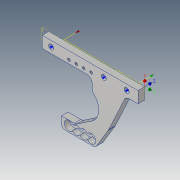
# Autodesk Inventor part: Extruder bracket
Saved by Autodesk Inventor 2019 (Build 230136000, 136)
## iProperties
Created: 2018-10-20
Part Number: Extruder bracket
Material: Aluminum 6061
Document SubType Name: Modeling
Designer: LillaHunden
Density: 2.7 g/cm^3
Appearance: Aluminum - Flat
Mass: 27.8066 g
Surface Area: 65.7368 cm^2
Volume: 10.2987 cm^3
Author: LillaHunden
Autodesk Inventor part; units mm, degrees
ref_plane "YZ Plane" through (0, 0, 0) normal (1, 0, 0) x (0, 1, 0)
ref_plane "XZ Plane" through (0, 0, 0) normal (0, 1, 0) x (-1, 0, 0)
ref_plane "XY Plane" through (0, 0, 0) normal (0, 0, 1) x (1, 0, 0)
sketch "Sketch3" plane through (0, 0, 0) normal (0, 0, 1) x (1, 0, 0)
  line L0 (-29.6423, -32.0618) -> (11.629, -32.0618)
  line L1 (11.629, -32.0618) -> (11.629, 19.8316)
  line L2 (11.629, 19.8316) -> (37.4023, 19.8316)
  line L3 (37.4023, 19.8316) -> (37.4023, 29.8316)
  line L4 (37.4023, 29.8316) -> (-52.693, 29.8316)
  line L5 (-52.693, 29.8316) -> (-52.693, 19.8316)
  line L6 (-52.693, 19.8316) -> (-2.6589, 19.8316)
  line L7 (-2.6589, 19.8316) -> (-2.6589, -22.8391)
  line L8 (-2.6589, -22.8391) -> (-29.6423, -22.8391)
  line L9 (-29.6423, -22.8391) -> (-29.6423, -32.0618)
  line L10 (37.4023, 19.8316) -> (-46.3977, 19.8316) projected
  point P0 (0, 0)
  constraints: 20 end point, 9 perpendicular, 1 horizontal, 1 horizontal alignment, 1 point on line
extrude "Extrusion3" add sketch "Sketch3" along normal blind 6
sketch "Sketch4" plane through (0, 0, 6) normal (0, 0, 1) x (1, 0, 0)
  circle A0 centre (-10.7483, -2.0987) radius 3.15 construction
  circle A1 centre (-10.7483, -2.0987) radius 13.7506
  point P0 (0, 0)
  constraints: 1 centre point, 1 coincident
extrude "Extrusion4" cut sketch "Sketch4" against normal through all
sketch "Sketch5" plane through (0, 0, 0) normal (0, 0, -1) x (-1, 0, 0)
  line L0 (-11.629, -32.0618) -> (-11.629, 19.8316) projected
  line L1 (-11.629, -12.8203) -> (-26.7273, 19.8316)
  line L2 (-11.629, 19.8316) -> (-37.4023, 19.8316) projected
  point P0 (0, 0)
  constraints: 2 end point, 2 point on line
extrude "Extrusion5" add sketch "Sketch5" against normal up to surface (6 mm away)
sketch "Sketch6" plane through (0, 0, 6) normal (0, 0, 1) x (1, 0, 0)
  line L0 (-2.6589, -22.8391) -> (-29.6423, -22.8391) projected
  line L1 (-2.6589, -13.218) -> (-2.6589, -22.8391) projected
  line L2 (-16.9254, -22.8391) -> (-2.6589, -13.218)
  point P0 (0, 0)
  constraints: 2 end point, 1 point on line
ref_plane "Work Plane1" through (-29.6423, -32.0618, 0) normal (0, 0, 1) x (1, 0, 0)
extrude "Extrusion6" add sketch "Sketch6" against normal up to surface (6 mm away)
sketch "Sketch7" plane through (0, 0, 0) normal (0, 0, -1) x (-1, 0, 0)
  line L0 (29.6423, -32.0618) -> (-11.629, -32.0618) projected
  line L1 (0, -32.0618) -> (-11.629, -12.8203)
  line L2 (-11.629, -32.0618) -> (-11.629, -12.8203) projected
  point P0 (0, 0)
  constraints: 2 end point, 1 point on line
extrude "Extrusion7" cut sketch "Sketch7" against normal through all
fillet "Fillet1" radius 5 6 edges at (-16.9254, -22.8391, 3) (-2.6589, -13.218, 3) (11.629, -12.8203, 3) (26.7273, 19.8316, 3) (-2.6589, 9.0207, 3) (-2.6589, 19.8316, 3)
fillet "Fillet2" radius 3 1 edges at (-29.6423, -32.0618, 3)
fillet "Fillet3" radius 3 1 edges at (0, -32.0618, 3)
sketch "Sketch8" plane through (0, 0, 0) normal (0, 0, -1) x (-1, 0, 0)
  line L0 (52.5977, 19.8316) -> (-37.4023, 19.8316) construction
  line L1 (-37.4023, 19.8316) -> (-37.4023, 29.8316) construction
  line L2 (52.5977, 29.8316) -> (-37.4023, 29.8316) construction
  line L3 (52.5977, 19.8316) -> (52.5977, 29.8316) construction
  line L4 (-37.4023, 19.8316) -> (-37.4023, 29.8316) construction
  line L5 (-37.4023, 24.8316) -> (52.693, 24.8316) construction
  line L6 (52.693, 29.8316) -> (52.693, 19.8316) construction
  point P0 (0, 0)
  point P1 (-27.4023, 24.8316)
  point P2 (-7.4023, 24.8316)
  point P3 (38.693, 24.8316)
  dimension "d20" = 10
  dimension "d21" = 14
  dimension "d23" = 20
  constraints: 3 point on line, 2 end point, 2 midpoint
  measures "d20" distance from line of L1 point (-27.402, 24.832)
  measures "d21" distance from line of L6 point (38.693, 24.832)
  measures "d23" distance of point (-7.402, 24.832) point (-27.402, 24.832)
sketch "Sketch9" plane through (0, 0, 0) normal (0, 0, -1) x (-1, 0, 0)
  point P0 (-27.4023, 24.8316)
  point P1 (-7.4023, 24.8316)
  point P2 (38.693, 24.8316)
hole "Hole1" at (27.4023, 24.8316, 0) at (7.4023, 24.8316, 0) at (-38.693, 24.8316, 0) direction (0, 0, 1) diameter 4.5 depth 6 counterbore diameter 8 counterbore depth 4
sketch "Sketch11" plane through (0, 0, 0) normal (0, 0, -1) x (-1, 0, 0)
  arc A0 (1.6423, 27.9382) -> (-1.3577, 24.9382) centre (1.6423, 24.9382) ccw construction
  line L0 (-1.3577, 12.9382) -> (-1.3577, 24.9382) construction
  line L1 (-1.3577, 12.9382) -> (29.6423, 12.9382) construction
  line L2 (29.6423, 24.9382) -> (29.6423, 12.9382) construction
  arc A1 (29.6423, 24.9382) -> (26.6423, 27.9382) centre (26.6423, 24.9382) ccw construction
  line L3 (1.6423, 27.9382) -> (26.6423, 27.9382) construction
  circle A2 centre (10.1423, 22.9382) radius 2.15 projected
  circle A3 centre (23.1423, 22.9382) radius 2.15 projected
  circle A4 centre (16.6423, 22.9382) radius 2.15 projected
  circle A5 centre (3.6423, 22.9382) radius 2.15 projected
  point P0 (0, 0)
  point P1 (16.6423, 22.9382)
  point P2 (10.1423, 22.9382)
  point P3 (3.6423, 22.9382)
hole "Hole4" at (-23.1423, 22.9382, 0) at (-16.6423, 22.9382, 0) at (-10.1423, 22.9382, 0) at (-3.6423, 22.9382, 0) direction (0, 0, 1) diameter 2.459 depth 8.8 thread size "M3x0.5" class "6H" standard "ISO Metric profile"
sketch "Sketch12" plane through (0, 0, 6) normal (0, 0, 1) x (1, 0, 0)
  point P0 (-3.6423, -27.0618)
  point P1 (-23.1423, -27.0618)
  point P2 (-16.6423, -27.0618)
  point P3 (-10.1423, -27.0618)
hole "Hole5" at (-3.6423, -27.0618, 6) at (-23.1423, -27.0618, 6) at (-16.6423, -27.0618, 6) at (-10.1423, -27.0618, 6) direction (0, 0, -1) diameter 4.5 depth 6 counterbore diameter 8 counterbore depth 4.6
sketch "Sketch13" plane through (-52.693, 19.8316, 0) normal (-1, 0, 0) x (0, 0, 1)
  line L0 (0, 10) -> (0, 0) projected
  line L1 (0, 0) -> (6, 0) projected
  line L2 (6, 10) -> (6, 0) projected
  line L3 (0, 10) -> (6, 10) projected
  point P0 (0, -19.8316)
ref_plane "Work Plane2" through (-46.5977, 19.8316, 6) normal (-1, 0, 0) x (0, 0, 1)
extrude "Extrusion8" cut sketch "Sketch13" against normal up to surface (6.0952 mm away)
chamfer "Chamfer1" distance 0.2 angle 45 20 edges at (-2.2661, 9.3844, 0) (2.9668, -3.0863, 0) (-9.1585, -17.6013, 0) (-16.9922, -22.6207, 0) (-24.0481, -22.8391, 0) (-2.6589, 13.0793, 0) (-4.1234, 18.3671, 0) (-27.1283, 19.8316, 0) (-29.6423, -25.9505, 0) (-28.7637, -31.1831, 0) (-14.1673, -32.0618, 0) (-0.2183, -31.6747, 0) (6.1806, -21.8353, 0) (11.6222, -12.8167, 0) (18.5654, 2.1804, 0) (27.2307, 19.0442, 0) (33.6631, 19.8316, 0) (37.4023, 24.8316, 0) (-4.5977, 29.8316, 0) (-46.5977, 24.8316, 0)
chamfer "Chamfer2" distance 0.1 angle 45 7 edges at (-38.693, 20.8316, 0) (-23.1423, 21.7087, 0) (-16.6423, 21.7087, 0) (-10.1423, 21.7087, 0) (-3.6423, 21.7087, 0) (7.4023, 20.8316, 0) (27.4023, 20.8316, 0)
body "Solid2"
